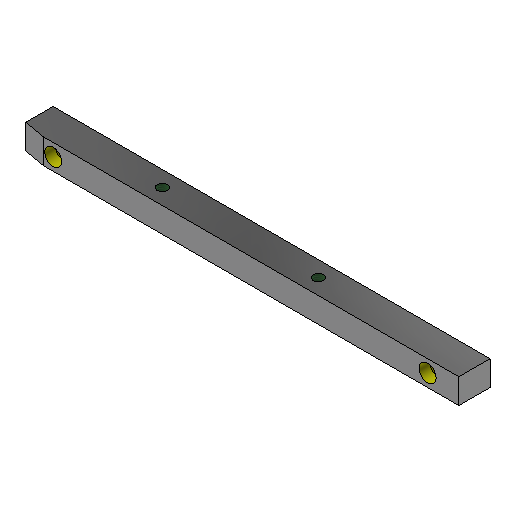
# Autodesk Inventor part: TL20240701-10120CV-015
Saved by Autodesk Inventor 2022.5 (Build 265521000, 521)
## iProperties
Category: FOLLOWER UNIT ASSY
Manager: 호상태
Company: 현대 트랜시스(대유)
Created: 2023-01-30
Part Number: TL20240701-10120CV-015
Project: SW PJT
Checked By: 김형민
Engr Approved By: 김시현
User Status: 2 x18
Material: S45C
Description: 0
Document SubType Name: Modeling
Mfg Approved By: 호상태
Designer: 박성규
Stock Number: 015
Mass: 645.041 g
Surface Area: 268.776 cm^2
Volume: 81.962 cm^3
Density: 7.87 g/cm^3
Appearance: Plating Chrome
DETAIL: Coveryor Assembly
M/C TITLE: MEa/NEa차종 시트조립라인
SPECIFICATION: TL20221201-000000CV-009
DocNumber: 221118_Standard_v1
Folder: .\
VDS_Category: 엔지니어링
Detail Description: Processed products
Title: PLATE GUIDE
Subject: SW차종 시트조립라인
Author: 박성규
Revision Number: A
Autodesk Inventor part; units mm, degrees
ref_plane "YZ Plane" through (0, 0, 0) normal (1, 0, 0) x (0, 1, 0)
ref_plane "XZ Plane" through (0, 0, 0) normal (0, 1, 0) x (-1, 0, 0)
ref_plane "XY Plane" through (0, 0, 0) normal (0, 0, 1) x (1, 0, 0)
sketch "스케치8" plane through (0, 0, 0) normal (0, 0, 1) x (1, 0, 0)
  line L0 (-140, 8) -> (140, 8)
  line L1 (140, 8) -> (140, -8)
  line L2 (140, -8) -> (-140, -8)
  line L3 (-140, -8) -> (-140, 8)
  line L4 (-140, 8) -> (140, -8) construction
  line L5 (140, 8) -> (-140, -8) construction
  point P0 (0, 0)
  dimension "d38" = 280
  dimension "d39" = 16
  constraints: 12 end point, 2 midpoint, 2 parallel, 1 horizontal, 1 perpendicular
  measures "d38" distance of L1.end L2.end
  measures "d39" distance of L0.end L1.end
extrude "돌출3" add sketch "스케치8" along normal blind 20
sketch "스케치9" plane through (0, 0, 20) normal (0, 0, 1) x (1, 0, 0)
  line L0 (-140, 8) -> (-140, -8) construction
  line L1 (140, -8) -> (140, 8) construction
  point P0 (0, 0)
  point P1 (-120, 0)
  point P2 (120, 0)
  dimension "d42" = 20
  dimension "d78" = 20
  constraints: 2 horizontal alignment
  measures "d42" distance from line of point (-120, 0) L0
  measures "d78" distance from line of L1 point (120, 0)
hole "구멍3" at (-120, 0, 20) at (120, 0, 20) direction (0, 0, -1) diameter 6.6 end through all counterbore diameter 11 counterbore depth 6.8 clearance for "Socket Head Cap Screw ISO 4762" size "M6" standard "ISO"
chamfer "모따기2" distance 14 angle 10 1 edges at (-140, 0, 20) measured on face at (-139.5, 0, 20)
sketch "Sketch11" plane through (-140, 8, 0) normal (0, 1, 0) x (1, 0, 0)
  line L0 (280, 0) -> (0, 0) projected
  line L1 (280, 0) -> (280, -20) projected
  point P0 (140, 0)
  point P1 (180, -10)
  point P2 (80, -10)
  dimension "d79" = 10
  dimension "d80" = 100
  dimension "d82" = 100
  constraints: 1 horizontal alignment
  measures "d79" distance from line of point (180, -10) L0
  measures "d80" distance from line of point (180, -10) L1
  measures "d82" distance of point (80, -10) point (180, -10)
hole "Hole5" at (40, 8, 10) at (-60, 8, 10) direction (0, -1, 0) diameter 6.647 end through all thread size "M8x1.25" class "6H" standard "TS profile"
